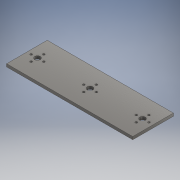
# Autodesk Inventor part: frontal2
Saved by Autodesk Inventor 2018 (Build 220112000, 112)
## iProperties
Created: 2019-04-02
Part Number: frontal2
Material: Acero, galvanizado
Document SubType Name: Modeling
Designer: Victor Hernandez
Density: 7.85 g/cm^3
Appearance: Galvanizado
Author: Victor Hernandez
Autodesk Inventor part; units mm, degrees
ref_plane "YZ Plane" through (0, 0, 0) normal (1, 0, 0) x (0, 1, 0)
ref_plane "XZ Plane" through (0, 0, 0) normal (0, 1, 0) x (-1, 0, 0)
ref_plane "XY Plane" through (0, 0, 0) normal (0, 0, 1) x (1, 0, 0)
sketch "Boceto1" plane through (0, 0, 0) normal (0, 0, 1) x (1, 0, 0)
  line L0 (-45, -14.5) -> (45, -14.5)
  line L1 (45, -14.5) -> (45, 14.5)
  line L2 (45, 14.5) -> (-45, 14.5)
  line L3 (-45, 14.5) -> (-45, -14.5)
  line L4 (45, -14.5) -> (-45, 14.5) construction
  circle A0 centre (0, 0) radius 2
  line L5 (0, 0) -> (4.5, 0) construction
  line L6 (0, 0) -> (4.5, 0)
  circle A1 centre (0, 4.5) radius 0.75
  circle A2 centre (4.5, 0) radius 0.75
  circle A3 centre (0, -4.5) radius 0.75
  circle A4 centre (-4.5, 0) radius 0.75
  circle A5 centre (-42, 0) radius 0.75
  circle A6 centre (-37.5, 0) radius 2
  circle A7 centre (-33, 0) radius 0.75
  circle A8 centre (-37.5, 4.5) radius 0.75
  circle A9 centre (-37.5, -4.5) radius 0.75
  circle A10 centre (37.5, 0) radius 2
  circle A11 centre (42, 0) radius 0.75
  circle A12 centre (37.5, 4.5) radius 0.75
  circle A13 centre (33, 0) radius 0.75
  circle A14 centre (37.5, -4.5) radius 0.75
  dimension "d0" = 90
  dimension "d1" = 29
  dimension "d2" = 4
  dimension "d8" = 1.5
  dimension "d9" = 1.5
  dimension "d10" = 1.5
  dimension "d11" = 1.5
  dimension "d23" = 4
  dimension "d25" = 1.5
  dimension "d28" = 1.5
  dimension "d29" = 1.5
  dimension "d35" = 4
  dimension "d36" = 1.5
  dimension "d37" = 1.5
  dimension "d38" = 1.5
  dimension "d39" = 1.5
  constraints: 15 centre point, 14 end point, 3 equal length, 2 coincident, 2 horizontal, 1 midpoint, 1 perpendicular
  measures "d0" distance of L2.end L1.end
  measures "d1" distance of L1.end L0.end
  measures "d2" diameter of A0
  measures "d8" diameter of A1
  measures "d9" diameter of A2
  measures "d10" diameter of A3
  measures "d11" diameter of A4
  measures "d23" diameter of A6
  measures "d25" diameter of A7
  measures "d28" diameter of A8
  measures "d29" diameter of A9
  measures "d35" diameter of A10
  measures "d36" diameter of A11
  measures "d37" diameter of A12
  measures "d38" diameter of A13
  measures "d39" diameter of A14
extrude "Extrusión1" add sketch "Boceto1" along normal blind 2
